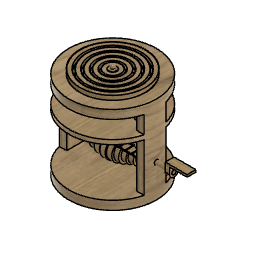
final project  v16 (Autodesk Fusion 360 design; units mm, degrees)
Autodesk Fusion 360 part; units mm, degrees
note: some values were not read from the file. Set by a fixed rule: which face or edge a step refers to.
sketch "holder sketch" plane through (0, 0, 0) normal (0, 0, 1) x (1, 0, 0) in component "Holder"
  line L0 (100, 0) -> (100, 25) construction
  line L1 (96.8246, 50) -> (-96.8246, 50)
  line L2 (-100, 50) -> (-100, 25) construction
  line L3 (-100, 0) -> (96.8246, 0)
  line L4 (-96.8246, 0) -> (-80, 0)
  line L5 (-80, 0) -> (-80, 50)
  line L6 (80, 0) -> (80, 50)
  line L7 (0, 0) -> (0, 50)
  line L8 (0, 25) -> (-100, 25)
  line L9 (0, 25) -> (100, 25)
  circle A0 centre (0, 25) radius 100
  line L10 (100, 50) -> (96.8246, 50) construction
  line L11 (100, 25) -> (100, 50) construction
  line L12 (96.8246, 0) -> (100, 0) construction
  line L13 (-100, 0) -> (-96.8246, 0) construction
  line L14 (-100, 25) -> (-100, 0) construction
  line L15 (-96.8246, 50) -> (-100, 50) construction
  line L16 (96.8246, 0) -> (80, 0)
  circle A1 centre (0, 25) radius 5
  circle A2 centre (14, 25) radius 5
  circle A3 centre (28, 25) radius 5
  circle A4 centre (42, 25) radius 5
  circle A5 centre (56, 25) radius 5
  circle A6 centre (70, 25) radius 5
  circle A7 centre (-14, 25) radius 5
  circle A8 centre (-28, 25) radius 5
  circle A9 centre (-42, 25) radius 5
  circle A10 centre (-56, 25) radius 5
  circle A11 centre (-70, 25) radius 5
  dimension "d1" = 20
  dimension "d2" = 200
  dimension "d3" = 50
  dimension "d18" = 70
  dimension "d19" = 0
  constraint perpendicular L1 L2
  constraint coincident L3 L4.end
  constraint coincident L1 L5.end
  constraint perpendicular L1 L5
  constraint coincident L3 L6.start
  constraint coincident L1 L6.end
  constraint perpendicular L1 L6
  constraint coincident L7.start origin
  constraint midpoint L7 L8.start
  constraint coincident L8.start L9.start
  constraint coincident L0.end A0
  constraint coincident A0 L1.start
  constraint coincident L1 L7.end
  constraint coincident A0 L3.end
  constraint perpendicular L0 L12
  constraint coincident A0 L4.start
  constraint perpendicular L1 L14
  constraint coincident A0 L1.end
  constraint concentric A0 A1
  constraint symmetric L7 A2 A7
  constraint symmetric L7 A3 A8
  constraint symmetric L7 A4 A9
  constraint symmetric L7 A5 A10
  constraint symmetric L7 A6 A11
  measures "d1" distance of L3.start L4.end
  measures "d2" distance of L0.start L3.start
  measures "d3" distance of L2.start L3.start
extrude "Extrude1" add sketch "holder sketch" along normal blind 20 makes body 1 in component "Holder"
extrude "Extrude2" add sketch "holder sketch" along normal blind 200 contours L1 L6 L9 A0 | L3 L6 L9 A0 L16 | L1 L5 L8 A0 | L3 L4 L5 L8 A0 bodies 1 in component "Holder"
extrude "Extrude3" add sketch "holder sketch" along normal blind 200 and the other way blind -180 bodies 1 in component "Holder"
extrude "Extrude4" add sketch "holder sketch" along normal blind 140 and the other way blind -130 bodies 1 in component "Holder"
extrude "Extrude5" cut sketch "holder sketch" along normal blind 225 and the other way blind -100 contours L7 L9 A1 | L7 L8 A1 | L9 A6 | L9 A6 | L7 L9 A1 | L7 L8 A1 | L8 A11 | L8 A11 | L9 A2 | L9 A2 | L8 A7 | L8 A7 | L9 A5 | L9 A5 | L8 A10 | L8 A10 | L9 A3 | L9 A3 | L8 A8 | L8 A8 | L9 A4 | L9 A4 | L8 A9 | L8 A9 bodies 1 in component "Holder"
sketch "hole holder sketch" plane through (80, 0, 0) normal (-1, 0, 0) x (0, -1, 0) in component "Holder"
  line L0 (0, 130) -> (-50, 130)
  line L1 (-50, 130) -> (-50, 20)
  line L2 (-50, 20) -> (0, 20)
  line L3 (0, 20) -> (0, 130)
  line L4 (-50, 130) -> (-50, 20) construction
  line L5 (0, 20) -> (0, 130) construction
  line L6 (-50, 75) -> (0, 75) construction
  circle A0 centre (-25, 75) radius 5
  dimension "d24" = 10
  constraint coincident L0.end L1.start
  constraint coincident L1.end L2.start
  constraint coincident L2.end L3.start
  constraint coincident L0.start L3.end
  constraint midpoint L4 L6.start
  constraint midpoint L5 L6.end
  constraint midpoint L6 A0.centre
  measures "d24" diameter of A0
extrude "Extrude6" cut sketch "hole holder sketch" along normal blind 225 and the other way blind 50 contours A0 bodies 1 in component "Holder"
sketch "axe&disks sketch" plane through (80, 0, 0) normal (-1, 0, 0) x (0, -1, 0) in component "Axe&disks"
  circle A0 centre (-25, 75) radius 5
  line L0 (0, 130) -> (-50, 130)
  line L1 (-50, 130) -> (-50, 20)
  line L2 (-50, 20) -> (0, 20)
  line L3 (0, 20) -> (0, 130)
  circle A1 centre (-25, 75) radius 5
  circle A2 centre (-25, 81.8988) radius 11.8988
  circle A3 centre (-25, 85) radius 15
  circle A4 centre (-25, 87.1115) radius 17.1115
  circle A5 centre (-25, 90) radius 20
  circle A6 centre (-25, 92.0859) radius 22.0859
  circle A7 centre (-25, 93.1028) radius 23.1028
  constraint concentric A0 A1
  constraint tangent A1 A2
  constraint tangent A2 A3
  constraint tangent A2 A4
  constraint tangent A1 A4
  constraint tangent A3 A5
  constraint tangent A4 A5
  constraint tangent A3 A6
  constraint tangent A1 A6
  constraint tangent A4 A7
extrude "Extrude1'" add sketch "axe&disks sketch" along normal blind 190 and the other way blind 60 separate body contours A0 A1 makes body 2 in component "Axe&disks"
move_face "OffsetFaces1" offset -0.3 4 faces at (-46.6667, 21.9092, 71.0697) (-46.6667, 29.4096, 72.643) (120, 22.0997, 70.9271) (120, 29.5199, 72.8622) on bodies 2 in component "Axe&disks"
sketch "handle sketch" plane through (80, 0, 0) normal (-1, 0, 0) x (0, -1, 0) in component "Handle"
  circle A0 centre (-25, 75) radius 10
  line L0 (-35, 75) -> (-15, 75)
  line L1 (-15, 75) -> (-15, 55)
  line L2 (-15, 55) -> (-35, 55)
  line L3 (-35, 55) -> (-35, 75)
  line L4 (-15, 55) -> (-35, 55)
  line L5 (-35, 55) -> (-35, 60)
  line L6 (-35, 60) -> (-15, 60)
  line L7 (-15, 60) -> (-15, 55)
  circle A1 centre (-25, 75) radius 5
  constraint horizontal L0
  constraint vertical L1
  constraint horizontal L2
  constraint vertical L3
  constraint coincident A0 L0.start
  constraint horizontal L4
  constraint vertical L5
  constraint horizontal L6
  constraint vertical L7
  constraint coincident L3 L5.end
  constraint concentric A0 A1
extrude "Extrude1''" add sketch "handle sketch" along normal blind -60 and the other way blind 50 separate body makes body 3 in component "Handle"
extrude "Extrude2'" add sketch "handle sketch" along normal blind -60 and the other way blind 100 contours L1 L2 L3 L4 L5 L6 L7 bodies 3 in component "Handle"
extrude "Extrude3'" cut sketch "handle sketch" along normal blind -67 and the other way blind 46 contours L0 A1 | L0 A1 bodies 3 in component "Handle"
move_face "OffsetFaces1'" offset -0.3 1 faces at (6.9652, -42.7894, 200) on bodies 1 in component "Holder"
sketch "ring 1 sketch" plane through (0, 0, 199.7) normal (0, 0, 1) x (-1, 0, 0) in component "ring 1"
  circle A0 centre (-42, -25) radius 5
  circle A1 centre (14, -25) radius 5
  circle A2 centre (70, -25) radius 5
  circle A3 centre (28, -25) radius 5
  circle A4 centre (-28, -25) radius 5
  circle A5 centre (-56, -25) radius 5
  circle A6 centre (0, -25) radius 5
  circle A7 centre (56, -25) radius 5
  circle A8 centre (42, -25) radius 5
  circle A9 centre (-14, -25) radius 5
  circle A10 centre (-70, -25) radius 5
  circle A11 centre (0, -25) radius 100
  circle A12 centre (0, -25) radius 75
  circle A13 centre (0, -25) radius 65
  circle A14 centre (70, -25) radius 3.5
  circle A15 centre (-70, -25) radius 3.5
  line L0 (75, -25) -> (-75, -25)
  line L1 (0, -25) -> (0, -35) construction
  line L2 (0, -25) -> (0, -15) construction
  line L3 (0, -25) -> (6, -25)
  line L4 (-14, -25) -> (-8, -25)
  line L5 (-28, -25) -> (-22, -25)
  line L6 (-42, -25) -> (-36, -25)
  line L7 (-56, -25) -> (-50, -25)
  line L8 (-70, -25) -> (-76, -25)
  line L9 (0, -5) -> (-76.2301, -5)
  line L10 (0, -45) -> (-76.2301, -45)
  line L11 (0, -5) -> (76.2301, -5)
  line L12 (0, -45) -> (76.2301, -45)
  line L13 (76.2301, -45) -> (76.2301, -5)
  line L14 (-76.2301, -45) -> (-76.2301, -5)
  line L15 (76.2301, -45) -> (64.2301, -45)
  line L16 (64.2301, -45) -> (64.2301, -5)
  line L17 (50, -45) -> (62, -45)
  line L18 (62, -45) -> (61.8466, -5)
  line L19 (50, -45) -> (50, -5)
  line L20 (48, -45) -> (36, -45)
  line L21 (36, -45) -> (36, -5)
  line L22 (48, -45) -> (48, -5)
  line L23 (34, -45) -> (22, -45)
  line L24 (22, -45) -> (22, -5)
  line L25 (34, -45) -> (34, -5)
  line L26 (20, -45) -> (8, -45)
  line L27 (8, -45) -> (8, -5)
  line L28 (0, -45) -> (6, -45)
  line L29 (6, -45) -> (6, -5)
  line L30 (-6, -45) -> (-6, -5)
  line L31 (-8, -45) -> (-8, -5)
  line L32 (-22, -45) -> (-22, -5)
  line L33 (-34, -45) -> (-34, -5)
  line L34 (-36, -45) -> (-36, -5)
  line L35 (-48, -45) -> (-48, -5)
  line L36 (-50, -45) -> (-50, -5)
  line L37 (-62, -45) -> (-61.8466, -5)
  line L38 (-64.2301, -45) -> (-64.2301, -5)
  line L39 (20, -45) -> (20, -5)
  line L40 (-20, -45) -> (-20, -5)
  circle A16 centre (70, -25) radius 2.5
  circle A17 centre (56, -25) radius 2.5
  circle A18 centre (42, -25) radius 2.5
  circle A19 centre (28, -25) radius 2.5
  circle A20 centre (14, -25) radius 2.5
  circle A21 centre (0, -25) radius 2.5
  circle A22 centre (-70, -25) radius 2.5
  circle A23 centre (-56, -25) radius 2.5
  circle A24 centre (-42, -25) radius 2.5
  circle A25 centre (-28, -25) radius 2.5
  circle A26 centre (-14, -25) radius 2.5
  circle A27 centre (0, -25) radius 2.5
  dimension "d91" = 7
  dimension "d92" = 7
  dimension "d332" = 12
  dimension "d333" = 12
  dimension "d334" = 12
  dimension "d335" = 12
  dimension "d336" = 12
  dimension "d337" = 6
  dimension "d363" = 5
  dimension "d364" = 5
  dimension "d365" = 5
  dimension "d366" = 5
  dimension "d367" = 5
  dimension "d368" = 5
  constraint concentric A6 A12
  constraint tangent A10 A12
  constraint concentric A12 A13
  constraint tangent A10 A13
  constraint concentric A2 A14
  constraint concentric A10 A15
  constraint coincident A2 L0.start
  constraint coincident A12 L0.end
  constraint coincident A10 L0.end
  constraint horizontal L0
  constraint coincident A6.centre A11.centre
  constraint perpendicular L0 L1
  constraint perpendicular L0 L2
  constraint coincident L0 L3.end
  constraint perpendicular L1 L3
  constraint coincident A9.centre L4.start
  constraint coincident L0 L4.end
  constraint coincident A4.centre L5.start
  constraint coincident L0 L5.end
  constraint coincident A0.centre L6.start
  constraint coincident L0 L6.end
  constraint coincident A5.centre L7.start
  constraint coincident L0 L7.end
  constraint coincident A10.centre A15.centre
  constraint coincident L0 L8.end
  constraint symmetric L0 L9.start L10.start
  constraint symmetric L0 L9.end L10.end
  constraint symmetric L1 L9.start L11.start
  constraint symmetric L1 L9.end L11.end
  constraint symmetric L1 L10.start L12.start
  constraint symmetric L1 L10.end L12.end
  constraint coincident L12 L17.start
  constraint coincident L12 L20.start
  constraint coincident L12 L23.start
  constraint coincident L12 L26.start
  constraint perpendicular L11 L13
  constraint coincident L12 L15.end
  constraint coincident L11 L16.end
  constraint perpendicular L11 L16
  constraint coincident L11 L18.end
  constraint coincident A13 L18.end
  constraint coincident L11 L19.end
  constraint perpendicular L11 L19
  constraint coincident L11 L21.end
  constraint perpendicular L11 L21
  constraint coincident L11 L22.end
  constraint perpendicular L11 L22
  constraint coincident L12 L23.end
  constraint coincident L11 L24.end
  constraint perpendicular L11 L24
  constraint coincident L11 L25.end
  constraint perpendicular L11 L25
  constraint coincident L12 L26.end
  constraint coincident L11 L27.end
  constraint perpendicular L11 L27
  constraint coincident L11 L29.end
  constraint perpendicular L11 L29
  constraint symmetric L2 L17.start L36.start
  constraint symmetric L2 L20.start L35.start
  constraint symmetric L2 L23.start L33.start
  constraint symmetric L2 L15.end L38.start
  constraint symmetric L2 L16.end L38.end
  constraint symmetric L2 L17.end L37.start
  constraint symmetric L2 L18.end L37.end
  constraint symmetric L2 L19.end L36.end
  constraint symmetric L2 L20.end L34.start
  constraint symmetric L2 L21.end L34.end
  constraint symmetric L2 L22.end L35.end
  constraint symmetric L2 L23.end L32.start
  constraint symmetric L2 L24.end L32.end
  constraint symmetric L2 L25.end L33.end
  constraint symmetric L2 L26.end L31.start
  constraint symmetric L2 L27.end L31.end
  constraint symmetric L2 L28.end L30.start
  constraint symmetric L2 L29.end L30.end
  constraint coincident L11 L39.end
  constraint perpendicular L11 L39
  constraint symmetric L1 L26.start L40.start
  constraint symmetric L1 L39.end L40.end
  constraint concentric A14 A16
  constraint concentric A7 A17
  constraint concentric A8 A18
  constraint concentric A3 A19
  constraint concentric A1 A20
  constraint concentric A13 A21
  constraint symmetric L2 A16 A22
  constraint symmetric L2 A17 A23
  constraint symmetric L2 A18 A24
  constraint symmetric L2 A19 A25
  constraint symmetric L2 A20 A26
  constraint symmetric L2 A21 A27
  measures "d91" diameter of A14
  measures "d92" diameter of A15
  measures "d332" distance of L12.end L15.end
  measures "d333" distance of L17.start L17.end
  measures "d334" distance of L20.start L20.end
  measures "d335" distance of L23.start L23.end
  measures "d336" distance of L26.start L26.end
  measures "d337" distance of L10.start L28.end
  measures "d363" diameter of A16
  measures "d364" diameter of A17
  measures "d365" diameter of A18
  measures "d366" diameter of A19
  measures "d367" diameter of A20
  measures "d368" diameter of A21
extrude "Extrude1'''" add sketch "ring 1 sketch" along normal blind 10 separate body contours A13 L10 L37 | A12 A13 L10 L12 L15 L17 | A12 A13 L9 L11 | A13 L9 L38 | A13 L10 L37 L38 | A13 L12 L17 L18 | A13 L11 L16 | A10 A12 A13 L9 L38 | A10 A12 A13 L10 L38 | A13 L12 L16 L18 | A2 A12 A13 L11 L16 | A10 A15 L0 L8 | A10 A15 L0 L8 | A2 A12 A13 L12 L15 L16 | A2 A14 L0 | A2 A14 L0 | A15 L0 L8 A22 | A15 L0 L8 A22 | A14 L0 A16 | A14 L0 A16 | L0 L8 A22 | L0 L8 A22 | L0 A16 | L0 A16 makes body 4 in component "ring 1"
extrude "Extrude2''" add sketch "ring 1 sketch" against normal blind 117 contours A15 L0 L8 A22 | A15 L0 L8 A22 | A14 L0 A16 | A14 L0 A16 | L0 L8 A22 | L0 L8 A22 | L0 A16 | L0 A16 bodies 4 in component "ring 1"
sketch "ring 2 sketch" plane through (0, 0, 199.4) normal (0, 0, 1) x (-1, 0, 0) in component "ring 2"
  circle A0 centre (-42, -25) radius 5
  circle A1 centre (14, -25) radius 5
  circle A2 centre (70, -25) radius 5
  circle A3 centre (28, -25) radius 5
  circle A4 centre (-28, -25) radius 5
  circle A5 centre (-56, -25) radius 5
  circle A6 centre (0, -25) radius 5
  circle A7 centre (56, -25) radius 5
  circle A8 centre (42, -25) radius 5
  circle A9 centre (-14, -25) radius 5
  circle A10 centre (-70, -25) radius 5
  circle A11 centre (0, -25) radius 100
  circle A12 centre (0, -25) radius 61
  circle A13 centre (0, -25) radius 51
  circle A14 centre (56, -25) radius 3.5
  circle A15 centre (-56, -25) radius 3.5
  dimension "d97" = 7
  dimension "d98" = 7
  constraint concentric A6 A12
  constraint tangent A5 A12
  constraint concentric A12 A13
  constraint tangent A5 A13
  constraint concentric A7 A14
  constraint concentric A5 A15
  measures "d97" diameter of A14
  measures "d98" diameter of A15
extrude "Extrude1''''" add sketch "ring 2 sketch" along normal blind 10 separate body contours A5 | A5 A7 A12 A13 | A5 A7 A12 A13 | A7 | A14 | A15 makes body 5 in component "ring 2"
extrude "Extrude2'''" add sketch "ring 2 sketch" against normal blind 116.7 contours A14 | A15 bodies 5 in component "ring 2"
sketch "ring 3 sketch" plane through (0, 0, 199.4) normal (0, 0, 1) x (-1, 0, 0) in component "ring 3"
  circle A0 centre (-42, -25) radius 5
  circle A1 centre (14, -25) radius 5
  circle A2 centre (70, -25) radius 5
  circle A3 centre (28, -25) radius 5
  circle A4 centre (-28, -25) radius 5
  circle A5 centre (-56, -25) radius 5
  circle A6 centre (0, -25) radius 5
  circle A7 centre (56, -25) radius 5
  circle A8 centre (42, -25) radius 5
  circle A9 centre (-14, -25) radius 5
  circle A10 centre (-70, -25) radius 5
  circle A11 centre (0, -25) radius 100
  circle A12 centre (0, -25) radius 47
  circle A13 centre (0, -25) radius 37
  circle A14 centre (42, -25) radius 3.5
  circle A15 centre (-42, -25) radius 3.5
  dimension "d103" = 7
  dimension "d104" = 7
  constraint concentric A6 A12
  constraint tangent A0 A12
  constraint concentric A12 A13
  constraint tangent A0 A13
  constraint concentric A8 A14
  constraint concentric A0 A15
  measures "d103" diameter of A14
  measures "d104" diameter of A15
extrude "Extrude1'''''" add sketch "ring 3 sketch" along normal blind 10 separate body contours A0 | A0 A8 A12 A13 | A0 A8 A12 A13 | A8 | A14 | A15 makes body 6 in component "ring 3"
extrude "Extrude2''''" add sketch "ring 3 sketch" against normal blind 116.7 contours A14 | A15 bodies 6 in component "ring 3"
sketch "ring 4 sketch" plane through (0, 0, 199.4) normal (0, 0, 1) x (-1, 0, 0) in component "ring 4"
  circle A0 centre (-42, -25) radius 5
  circle A1 centre (14, -25) radius 5
  circle A2 centre (70, -25) radius 5
  circle A3 centre (28, -25) radius 5
  circle A4 centre (-28, -25) radius 5
  circle A5 centre (-56, -25) radius 5
  circle A6 centre (0, -25) radius 5
  circle A7 centre (56, -25) radius 5
  circle A8 centre (42, -25) radius 5
  circle A9 centre (-14, -25) radius 5
  circle A10 centre (-70, -25) radius 5
  circle A11 centre (0, -25) radius 100
  circle A12 centre (0, -25) radius 33
  circle A13 centre (0, -25) radius 23
  circle A14 centre (28, -25) radius 3.5
  circle A15 centre (-28, -25) radius 3.5
  dimension "d109" = 7
  dimension "d110" = 7
  constraint concentric A6 A12
  constraint tangent A4 A12
  constraint concentric A12 A13
  constraint tangent A4 A13
  constraint concentric A3 A14
  constraint concentric A4 A15
  measures "d109" diameter of A14
  measures "d110" diameter of A15
extrude "Extrude1''''''" add sketch "ring 4 sketch" along normal blind 10 separate body contours A3 | A3 A4 A12 A13 | A3 A4 A12 A13 | A4 | A14 | A15 makes body 7 in component "ring 4"
extrude "Extrude2'''''" add sketch "ring 4 sketch" against normal blind 116.7 contours A14 | A15 bodies 7 in component "ring 4"
sketch "ring 5 sketch" plane through (0, 0, 199.4) normal (0, 0, 1) x (-1, 0, 0) in component "ring 5"
  circle A0 centre (-42, -25) radius 5
  circle A1 centre (14, -25) radius 5
  circle A2 centre (70, -25) radius 5
  circle A3 centre (28, -25) radius 5
  circle A4 centre (-28, -25) radius 5
  circle A5 centre (-56, -25) radius 5
  circle A6 centre (0, -25) radius 5
  circle A7 centre (56, -25) radius 5
  circle A8 centre (42, -25) radius 5
  circle A9 centre (-14, -25) radius 5
  circle A10 centre (-70, -25) radius 5
  circle A11 centre (0, -25) radius 100
  circle A12 centre (0, -25) radius 19
  circle A13 centre (0, -25) radius 9
  circle A14 centre (14, -25) radius 3.5
  circle A15 centre (-14, -25) radius 3.5
  dimension "d115" = 7
  dimension "d116" = 7
  constraint concentric A6 A12
  constraint tangent A9 A12
  constraint concentric A12 A13
  constraint tangent A9 A13
  constraint concentric A1 A14
  constraint concentric A9 A15
  measures "d115" diameter of A14
  measures "d116" diameter of A15
extrude "Extrude1'''''''" add sketch "ring 5 sketch" along normal blind 10 separate body contours A1 | A1 A9 A12 A13 | A1 A9 A12 A13 | A9 | A14 | A15 makes body 8 in component "ring 5"
extrude "Extrude2''''''" add sketch "ring 5 sketch" against normal blind 116.7 contours A14 | A15 bodies 8 in component "ring 5"
sketch "central ring (6) sketch" plane through (0, 0, 199.4) normal (0, 0, 1) x (-1, 0, 0) in component "ring 6-central"
  circle A0 centre (-42, -25) radius 5
  circle A1 centre (14, -25) radius 5
  circle A2 centre (70, -25) radius 5
  circle A3 centre (28, -25) radius 5
  circle A4 centre (-28, -25) radius 5
  circle A5 centre (-56, -25) radius 5
  circle A6 centre (0, -25) radius 5
  circle A7 centre (56, -25) radius 5
  circle A8 centre (42, -25) radius 5
  circle A9 centre (-14, -25) radius 5
  circle A10 centre (-70, -25) radius 5
  circle A11 centre (0, -25) radius 100
  circle A12 centre (0, -25) radius 5
  circle A13 centre (0, -25) radius 3.5
  dimension "d122" = 7
  constraint concentric A6 A12
  constraint concentric A12 A13
  measures "d122" diameter of A13
extrude "Extrude1''''''''" add sketch "central ring (6) sketch" along normal blind -117 and the other way blind -15 separate body contours A13 makes body 9 in component "ring 6-central"
sphere "SpherePrimitive1" add diameter 10 placed x (-1, 0, 0) y (0, -1, 0) z (0, 0, 1) at (0, 25, 214.4) bodies 9 in component "ring 6-central"
extrude "Extrude2'''''''" add sketch "axe&disks sketch" along normal blind 15 and the other way blind -4 separate body contours A0 A1 | A2 makes body 10 in component "Axe&disks"
extrude "Extrude3''" add sketch "axe&disks sketch" along normal blind 30 and the other way blind -18 separate body contours A0 A1 | A2 | A3 makes body 11 in component "Axe&disks"
extrude "Extrude4'" add sketch "axe&disks sketch" along normal blind 43.5 and the other way blind -32.5 separate body contours A0 A1 | A2 | A3 | A4 makes body 12 in component "Axe&disks"
extrude "Extrude5'" add sketch "axe&disks sketch" along normal blind 57.5 and the other way blind -46.5 separate body contours A0 A1 | A2 | A3 | A4 | A5 makes body 13 in component "Axe&disks"
extrude "Extrude6'" add sketch "axe&disks sketch" along normal blind 72 and the other way blind -60 separate body contours A0 A1 | A2 | A3 | A4 | A5 | A6 makes body 14 in component "Axe&disks"
extrude "Extrude8" add sketch "axe&disks sketch" along normal blind 155.5 and the other way blind -144.5 separate body contours A0 A1 | A2 makes body 15 in component "Axe&disks"
extrude "Extrude9" add sketch "axe&disks sketch" along normal blind 130.5 and the other way blind -141.5 separate body contours A0 A1 | A2 | A3 makes body 16 in component "Axe&disks"
extrude "Extrude10" add sketch "axe&disks sketch" along normal blind 128 and the other way blind -116 separate body contours A0 A1 | A2 | A3 | A4 makes body 17 in component "Axe&disks"
extrude "Extrude11" add sketch "axe&disks sketch" along normal blind 113.5 and the other way blind -102.5 separate body contours A0 A1 | A2 | A3 | A4 | A5 makes body 18 in component "Axe&disks"
extrude "Extrude12" add sketch "axe&disks sketch" along normal blind 100 and the other way blind -88 separate body contours A0 A1 | A2 | A3 | A4 | A5 | A6 makes body 19 in component "Axe&disks"
extrude "Extrude13" add sketch "axe&disks sketch" along normal blind 74 and the other way blind -86 separate body contours A0 A1 | A2 | A3 | A4 | A5 | A6 | A7 makes body 20 in component "Axe&disks"
extrude "Extrude5''" add sketch "ring 1 sketch" along normal blind -117 and the other way blind 120 separate body contours A13 L0 L38 | A10 A12 A13 L9 L38 | A13 L0 L38 | A10 A12 A13 L10 L38 | A2 A12 A13 L11 L16 | A13 L0 L16 | A10 A15 L0 L8 | A10 A15 L0 L8 | A12 L9 L10 L14 | A13 L0 L16 | A2 A12 A13 L12 L15 L16 | A2 A14 L0 | A2 A14 L0 | A12 L11 L12 L13 L15 | A15 L0 L8 A22 | A15 L0 L8 A22 | A14 L0 A16 | A14 L0 A16 | L0 L8 A22 | L0 L8 A22 | L0 A16 | L0 A16 makes body 21 at (-68.2301, 18.3333, 79.7) makes body 22 at (72.2301, 18.3333, 79.7) in component "ring 1"
extrude "Extrude4''" add sketch "ring 1 sketch" along normal blind -117 and the other way blind 120 separate body contours A5 A13 L0 L7 L10 L36 L37 | A5 L0 L7 L9 L36 L37 | A5 L0 L7 A23 | A5 L0 L7 A23 | L0 L7 A23 | L0 L7 A23 | A7 A13 L0 L12 L17 L18 L19 | A7 L0 L11 L18 L19 | A7 L0 A17 | A7 L0 A17 | L0 A17 | L0 A17 makes body 23 at (53.9994, 31.5083, 79.7) makes body 24 at (-53.9994, 31.5083, 79.7) in component "ring 2"
extrude "Extrude4'''" add sketch "ring 1 sketch" along normal blind -117 and the other way blind 120 separate body contours A0 L0 L6 A24 | A0 L0 L6 L10 L34 L35 | A0 L0 L6 L9 L34 L35 | A0 L0 L6 A24 | L0 L6 A24 | L0 L6 A24 | A8 L0 L12 L20 L21 L22 | A8 L0 L11 L21 L22 | A8 L0 A18 | A8 L0 A18 | L0 A18 | L0 A18 makes body 25 at (-40, 31.6667, 79.7) makes body 26 at (44, 18.3333, 79.7) in component "ring 3"
extrude "Extrude4''''" add sketch "ring 1 sketch" along normal blind -117 and the other way blind 120 separate body contours A4 L0 L5 L9 L32 L33 | A4 L0 L5 L10 L32 L33 | A4 L0 L5 A25 | A4 L0 L5 A25 | L0 L5 A25 | L0 L5 A25 | A3 L0 L12 L23 L24 L25 | A3 L0 L11 L24 L25 | A3 L0 A19 | A3 L0 A19 | L0 A19 | L0 A19 makes body 27 at (30, 31.6667, 79.7) makes body 28 at (-30, 18.3333, 79.7) in component "ring 4"
extrude "Extrude4'''''" add sketch "ring 1 sketch" along normal blind -117 and the other way blind 120 separate body contours A9 L0 L4 L10 L31 L40 | A9 L0 L4 L9 L31 L40 | A9 L0 L4 A26 | A9 L0 L4 A26 | L0 L4 A26 | L0 L4 A26 | A1 L0 L12 L26 L27 L39 | A1 L0 L11 L27 L39 | A1 L0 A20 | A1 L0 A20 | L0 A20 | L0 A20 makes body 29 at (-16, 31.6667, 79.7) makes body 30 at (16, 31.6667, 79.7) in component "ring 5"
extrude "Extrude3'''" add sketch "ring 1 sketch" along normal blind -117 and the other way blind 120 separate body contours A6 L0 L3 L10 L12 L28 L29 L30 | A6 L0 L3 L9 L11 L29 L30 | A6 L0 L3 A21 A27 | A6 L0 L3 A21 A27 | L0 L3 A21 A27 | L0 L3 A21 A27 makes body 31 in component "ring 6-central"
extrude "Extrude6''" add sketch "ring 1 sketch" along normal blind -107 and the other way blind 117 contours L0 L8 A22 | L0 L8 A22 | L0 A16 | L0 A16 bodies 21 22 in component "ring 1"
shell "Shell1" thickness 0.7 removed faces 2 at (-56.6886, 24.2579, 82.7) at (55.3114, 24.2579, 82.7) on bodies 5 in component "ring 2"
extrude "Extrude5'''" add sketch "ring 1 sketch" along normal blind -107 and the other way blind 117 contours L0 L7 A23 | L0 L7 A23 | L0 A17 | L0 A17 bodies 23 24 in component "ring 2"
shell "Shell1'" thickness 0.7 removed faces 2 at (-41.4167, 24.4233, 82.7) at (41.2423, 23.9896, 82.7) on bodies 6 in component "ring 3"
extrude "Extrude5''''" add sketch "ring 1 sketch" along normal blind -107 and the other way blind 117 contours L0 L6 A24 | L0 L6 A24 | L0 A18 | L0 A18 bodies 25 26 in component "ring 3"
shell "Shell1''" thickness 0.7 removed faces 2 at (29.0511, 24.4938, 82.7) at (-26.9489, 24.4938, 82.7) on bodies 7 in component "ring 4"
extrude "Extrude5'''''" add sketch "ring 1 sketch" along normal blind -107 and the other way blind 117 contours L0 L5 A25 | L0 L5 A25 | L0 A19 | L0 A19 bodies 27 28 in component "ring 4"
shell "Shell4" thickness 0.7 removed faces 2 at (-69.2726, 26.5999, 82.7) at (70.7274, 26.5999, 82.7) on bodies 4 in component "ring 1"
shell "Shell1'''" thickness 0.7 removed faces 2 at (-15.0511, 24.8416, 82.7) at (12.8852, 25.3439, 82.7) on bodies 8 in component "ring 5"
extrude "Extrude5''''''" add sketch "ring 1 sketch" along normal blind -107 and the other way blind 117 contours L0 L4 A26 | L0 L4 A26 | L0 A20 | L0 A20 bodies 29 30 in component "ring 5"
shell "Shell1''''" thickness 0.7 removed faces 1 at (1.103, 24.1499, 82.4) on bodies 9 in component "ring 6-central"
extrude "Extrude4''''''" add sketch "ring 1 sketch" along normal blind -107 and the other way blind 117 contours L0 L3 A21 A27 | L0 L3 A21 A27 bodies 31 in component "ring 6-central"
component "Holder" placed x (1, 0, 0) y (0, 1, 0) z (0, 0, 1) at (0, 0, 0)
component "Axe&disks" placed x (1, 0, 0) y (0, -1, 0) z (0, 0, -1) at (0, 50, 150)
component "Handle" placed x (1, 0, 0) y (0, -1, 0) z (0, 0, -1) at (0, 50, 150)
component "ring 1" placed x (1, 0, 0) y (0, 1, 0) z (0, 0, 1) at (0, 0, 0.3)
component "ring 2" placed x (1, 0, 0) y (0, 1, 0) z (0, 0, 1) at (0, 0, 0.3)
component "ring 3" placed x (1, 0, 0) y (0, 1, 0) z (0, 0, 1) at (0, 0, 0.3)
component "ring 4" placed x (1, 0, 0) y (0, 1, 0) z (0, 0, 1) at (0, 0, 0.3)
component "ring 5" placed x (1, 0, 0) y (0, 1, 0) z (0, 0, 1) at (0, 0, 0.3)
component "ring 6-central" placed x (1, 0, 0) y (0, 1, 0) z (0, 0, 1) at (0, 0, 0.3)
named bodies: "holder body", "axe body", "handle body", "ring 1 body", "ring 2 body", "ring 3 body", "ring 4 body", "ring 5 body", "central ring (6) body", "disk 1 body", "disk 2 body", "disk 3 body", "disk 4 body", "disk 5 body", "disk 1 body 2", "disk 2 body 2", "disk 3 body 2", "disk 4 body 2", "disk 5 body 2", "disk 6 central body", "ring 1 base 1 body", "ring 1 base 2 body", "ring 2 base 1 body", "ring 2 base 2 body", "ring 3 base 1 body", "ring 3 base 2 body", "ring 4 base 1 body", "ring 4 base 2 body", "ring 5 base 1 body", "ring 5 base 2 body", "ring 6 base body"
